Autodesk Inventor part; units mm, degrees
(part 2 of 2)
sketch "Sketch2" plane through (0, 0, 0.5) normal (0, 0, 1) x (1, 0, 0)
  line L0 (260.2818, -61.0161) -> (260.2818, -88.6954) projected
  line L1 (260.2818, -88.6954) -> (269.6798, -88.6954) projected
  line L2 (269.6798, -88.6954) -> (269.6798, -107.7454) projected
  line L3 (269.6798, -107.7454) -> (274.7598, -107.7454) projected
  line L4 (274.7598, -107.7454) -> (274.7598, -126.7954) projected
  line L5 (274.7598, -126.7954) -> (265.1048, -126.7954) projected
  line L6 (265.1048, -126.7954) -> (265.1048, -148.1602) projected
  line L7 (265.1048, -148.1602) -> (272.1064, -148.1602) projected
  line L8 (272.1064, -148.1602) -> (272.1064, -165) projected
  line L9 (272.1064, -165) -> (327.9413, -165) projected
  line L10 (327.9413, -165) -> (327.9413, -146) construction
  line L11 (327.9413, -146) -> (405.2108, -146) projected
  line L12 (405.2108, -146) -> (405.2108, -165) projected
  line L13 (405.2108, -165) -> (490, -165) projected
  line L14 (490, -165) -> (490, -69.6056) projected
  line L15 (490, -69.6056) -> (316.8693, -69.6056) projected
  line L16 (316.8693, -69.6056) -> (316.8693, -40) construction
  line L17 (316.8693, -40) -> (269.5528, -40) construction
  line L18 (269.5528, -40) -> (269.5528, -61.0161) construction
  line L19 (269.5528, -61.0161) -> (260.2818, -61.0161) projected
  line L20 (318.1433, -116.8724) -> (330.6708, -116.8724) projected
  line L21 (330.6708, -116.8724) -> (330.6708, -122.8724) projected
  line L22 (330.6708, -122.8724) -> (318.1433, -122.8724) projected
  line L23 (318.1433, -122.8724) -> (318.1433, -120.8724) projected
  line L24 (318.1433, -120.8724) -> (316.6433, -120.8724) projected
  line L25 (316.6433, -120.8724) -> (316.6433, -118.8724) projected
  line L26 (316.6433, -118.8724) -> (318.1433, -118.8724) projected
  line L27 (318.1433, -118.8724) -> (318.1433, -116.8724) projected
  line L28 (471.9563, -154.774) -> (484.4563, -154.774) projected
  line L29 (484.4563, -154.774) -> (484.4563, -160.774) projected
  line L30 (484.4563, -160.774) -> (471.9563, -160.774) projected
  line L31 (471.9563, -160.774) -> (471.9563, -158.774) projected
  line L32 (471.9563, -158.774) -> (470.4563, -158.774) projected
  line L33 (470.4563, -158.774) -> (470.4563, -156.774) projected
  line L34 (470.4563, -156.774) -> (471.9563, -156.774) projected
  line L35 (471.9563, -156.774) -> (471.9563, -154.774) projected
  line L36 (318.1433, -92.8724) -> (330.6708, -92.8724) projected
  line L37 (330.6708, -92.8724) -> (330.6708, -98.8724) projected
  line L38 (330.6708, -98.8724) -> (318.1433, -98.8724) projected
  line L39 (318.1433, -98.8724) -> (318.1433, -96.8724) projected
  line L40 (318.1433, -96.8724) -> (316.6433, -96.8724) projected
  line L41 (316.6433, -96.8724) -> (316.6433, -94.8724) projected
  line L42 (316.6433, -94.8724) -> (318.1433, -94.8724) projected
  line L43 (318.1433, -94.8724) -> (318.1433, -92.8724) projected
  circle A0 centre (265, -64.8616) radius 3.25 projected
  line L44 (471.7063, -138.7715) -> (485.7113, -138.7715) projected
  line L45 (485.7113, -138.7715) -> (485.7113, -152.7765) projected
  line L46 (485.7113, -152.7765) -> (471.7063, -152.7765) projected
  line L47 (471.7063, -152.7765) -> (471.7063, -138.7715) projected
  line L48 (452.6563, -148.3679) -> (466.6613, -148.3679) projected
  line L49 (466.6613, -148.3679) -> (466.6613, -162.3729) projected
  line L50 (466.6613, -162.3729) -> (452.6563, -162.3729) projected
  line L51 (452.6563, -162.3729) -> (452.6563, -148.3679) projected
  line L52 (424.2083, -148.3679) -> (438.2133, -148.3679) projected
  line L53 (438.2133, -148.3679) -> (438.2133, -162.3729) projected
  line L54 (438.2133, -162.3729) -> (424.2083, -162.3729) projected
  line L55 (424.2083, -162.3729) -> (424.2083, -148.3679) projected
  line L56 (452.6563, -129.2195) -> (466.6613, -129.2195) projected
  line L57 (466.6613, -129.2195) -> (466.6613, -143.2245) projected
  line L58 (466.6613, -143.2245) -> (452.6563, -143.2245) projected
  line L59 (452.6563, -143.2245) -> (452.6563, -129.2195) projected
  line L60 (433.6063, -129.2195) -> (447.6113, -129.2195) projected
  line L61 (447.6113, -129.2195) -> (447.6113, -143.2245) projected
  line L62 (447.6113, -143.2245) -> (433.6063, -143.2245) projected
  line L63 (433.6063, -143.2245) -> (433.6063, -129.2195) projected
  line L64 (414.5563, -129.2195) -> (428.5613, -129.2195) projected
  line L65 (428.5613, -129.2195) -> (428.5613, -143.2245) projected
  line L66 (428.5613, -143.2245) -> (414.5563, -143.2245) projected
  line L67 (414.5563, -143.2245) -> (414.5563, -129.2195) projected
  line L68 (452.6563, -110.1695) -> (466.6613, -110.1695) projected
  line L69 (466.6613, -110.1695) -> (466.6613, -124.1745) projected
  line L70 (466.6613, -124.1745) -> (452.6563, -124.1745) projected
  line L71 (452.6563, -124.1745) -> (452.6563, -110.1695) projected
  line L72 (433.6063, -110.1695) -> (447.6113, -110.1695) projected
  line L73 (447.6113, -110.1695) -> (447.6113, -124.1745) projected
  line L74 (447.6113, -124.1745) -> (433.6063, -124.1745) projected
  line L75 (433.6063, -124.1745) -> (433.6063, -110.1695) projected
  line L76 (414.5563, -110.1695) -> (428.5613, -110.1695) projected
  line L77 (428.5613, -110.1695) -> (428.5613, -124.1745) projected
  line L78 (428.5613, -124.1745) -> (414.5563, -124.1745) projected
  line L79 (414.5563, -124.1745) -> (414.5563, -110.1695) projected
  line L80 (414.5563, -91.1195) -> (428.5613, -91.1195) projected
  line L81 (428.5613, -91.1195) -> (428.5613, -105.1245) projected
  line L82 (428.5613, -105.1245) -> (414.5563, -105.1245) projected
  line L83 (414.5563, -105.1245) -> (414.5563, -91.1195) projected
  line L84 (433.6063, -91.1195) -> (447.6113, -91.1195) projected
  line L85 (447.6113, -91.1195) -> (447.6113, -105.1245) projected
  line L86 (447.6113, -105.1245) -> (433.6063, -105.1245) projected
  line L87 (433.6063, -105.1245) -> (433.6063, -91.1195) projected
  line L88 (452.6563, -91.1195) -> (466.6613, -91.1195) projected
  line L89 (466.6613, -91.1195) -> (466.6613, -105.1245) projected
  line L90 (466.6613, -105.1245) -> (452.6563, -105.1245) projected
  line L91 (452.6563, -105.1245) -> (452.6563, -91.1195) projected
  line L92 (471.7063, -91.1195) -> (485.7113, -91.1195) projected
  line L93 (485.7113, -91.1195) -> (485.7113, -105.1245) projected
  line L94 (485.7113, -105.1245) -> (471.7063, -105.1245) projected
  line L95 (471.7063, -105.1245) -> (471.7063, -91.1195) projected
  line L96 (471.7063, -72.0695) -> (485.7113, -72.0695) projected
  line L97 (485.7113, -72.0695) -> (485.7113, -86.0745) projected
  line L98 (485.7113, -86.0745) -> (471.7063, -86.0745) projected
  line L99 (471.7063, -86.0745) -> (471.7063, -72.0695) projected
  line L100 (452.6563, -72.0695) -> (466.6613, -72.0695) projected
  line L101 (466.6613, -72.0695) -> (466.6613, -86.0745) projected
  line L102 (466.6613, -86.0745) -> (452.6563, -86.0745) projected
  line L103 (452.6563, -86.0745) -> (452.6563, -72.0695) projected
  line L104 (433.6063, -72.0695) -> (447.6113, -72.0695) projected
  line L105 (447.6113, -72.0695) -> (447.6113, -86.0745) projected
  line L106 (447.6113, -86.0745) -> (433.6063, -86.0745) projected
  line L107 (433.6063, -86.0745) -> (433.6063, -72.0695) projected
  line L108 (414.5563, -72.0695) -> (428.5613, -72.0695) projected
  line L109 (428.5613, -72.0695) -> (428.5613, -86.0745) projected
  line L110 (428.5613, -86.0745) -> (414.5563, -86.0745) projected
  line L111 (414.5563, -86.0745) -> (414.5563, -72.0695) projected
  line L112 (381.1515, -72.1031) -> (395.1565, -72.1031) projected
  line L113 (395.1565, -72.1031) -> (395.1565, -86.1081) projected
  line L114 (395.1565, -86.1081) -> (381.1515, -86.1081) projected
  line L115 (381.1515, -86.1081) -> (381.1515, -72.1031) projected
  line L116 (352.5555, -72.1031) -> (366.5605, -72.1031) projected
  line L117 (366.5605, -72.1031) -> (366.5605, -86.1081) projected
  line L118 (366.5605, -86.1081) -> (352.5555, -86.1081) projected
  line L119 (352.5555, -86.1081) -> (352.5555, -72.1031) projected
  line L120 (366.8775, -110.2171) -> (380.8825, -110.2171) projected
  line L121 (380.8825, -110.2171) -> (380.8825, -124.2221) projected
  line L122 (380.8825, -124.2221) -> (366.8775, -124.2221) projected
  line L123 (366.8775, -124.2221) -> (366.8775, -110.2171) projected
  line L124 (385.9275, -129.2671) -> (399.9325, -129.2671) projected
  line L125 (399.9325, -129.2671) -> (399.9325, -143.2721) projected
  line L126 (399.9325, -143.2721) -> (385.9275, -143.2721) projected
  line L127 (385.9275, -143.2721) -> (385.9275, -129.2671) projected
  line L128 (366.8775, -129.2671) -> (380.8825, -129.2671) projected
  line L129 (380.8825, -129.2671) -> (380.8825, -143.2721) projected
  line L130 (380.8825, -143.2721) -> (366.8775, -143.2721) projected
  line L131 (366.8775, -143.2721) -> (366.8775, -129.2671) projected
  line L132 (347.8275, -129.2671) -> (361.8325, -129.2671) projected
  line L133 (361.8325, -129.2671) -> (361.8325, -143.2721) projected
  line L134 (361.8325, -143.2721) -> (347.8275, -143.2721) projected
  line L135 (347.8275, -143.2721) -> (347.8275, -129.2671) projected
  line L136 (302.9363, -148.3679) -> (316.9413, -148.3679) projected
  line L137 (316.9413, -148.3679) -> (316.9413, -162.3729) projected
  line L138 (316.9413, -162.3729) -> (302.9363, -162.3729) projected
  line L139 (302.9363, -162.3729) -> (302.9363, -148.3679) projected
  line L140 (279.0603, -148.3679) -> (293.0653, -148.3679) projected
  line L141 (293.0653, -148.3679) -> (293.0653, -162.3729) projected
  line L142 (293.0653, -162.3729) -> (279.0603, -162.3729) projected
  line L143 (279.0603, -162.3729) -> (279.0603, -148.3679) projected
  line L144 (303.4443, -129.3179) -> (317.4493, -129.3179) projected
  line L145 (317.4493, -129.3179) -> (317.4493, -143.3229) projected
  line L146 (317.4493, -143.3229) -> (303.4443, -143.3229) projected
  line L147 (303.4443, -143.3229) -> (303.4443, -129.3179) projected
  line L148 (267.6303, -129.3179) -> (281.6353, -129.3179) projected
  line L149 (281.6353, -129.3179) -> (281.6353, -143.3229) projected
  line L150 (281.6353, -143.3229) -> (267.6303, -143.3229) projected
  line L151 (267.6303, -143.3229) -> (267.6303, -129.3179) projected
  line L152 (296.3323, -110.2679) -> (310.3373, -110.2679) projected
  line L153 (310.3373, -110.2679) -> (310.3373, -124.2729) projected
  line L154 (310.3373, -124.2729) -> (296.3323, -124.2729) projected
  line L155 (296.3323, -124.2729) -> (296.3323, -110.2679) projected
  line L156 (277.2823, -110.2679) -> (291.2873, -110.2679) projected
  line L157 (291.2873, -110.2679) -> (291.2873, -124.2729) projected
  line L158 (291.2873, -124.2729) -> (277.2823, -124.2729) projected
  line L159 (277.2823, -124.2729) -> (277.2823, -110.2679) projected
  line L160 (317.6433, -100.8949) -> (331.6483, -100.8949) projected
  line L161 (331.6483, -100.8949) -> (331.6483, -114.8999) projected
  line L162 (331.6483, -114.8999) -> (317.6433, -114.8999) projected
  line L163 (317.6433, -114.8999) -> (317.6433, -100.8949) projected
  line L164 (291.2523, -91.2179) -> (305.2573, -91.2179) projected
  line L165 (305.2573, -91.2179) -> (305.2573, -105.2229) projected
  line L166 (305.2573, -105.2229) -> (291.2523, -105.2229) projected
  line L167 (291.2523, -105.2229) -> (291.2523, -91.2179) projected
  line L168 (272.2023, -91.2179) -> (286.2073, -91.2179) projected
  line L169 (286.2073, -91.2179) -> (286.2073, -105.2229) projected
  line L170 (286.2073, -105.2229) -> (272.2023, -105.2229) projected
  line L171 (272.2023, -105.2229) -> (272.2023, -91.2179) projected
  line L172 (319.9543, -72.1679) -> (333.9593, -72.1679) projected
  line L173 (333.9593, -72.1679) -> (333.9593, -86.1729) projected
  line L174 (333.9593, -86.1729) -> (319.9543, -86.1729) projected
  line L175 (319.9543, -86.1729) -> (319.9543, -72.1679) projected
  line L176 (300.9043, -72.1679) -> (314.9093, -72.1679) projected
  line L177 (314.9093, -72.1679) -> (314.9093, -86.1729) projected
  line L178 (314.9093, -86.1729) -> (300.9043, -86.1729) projected
  line L179 (300.9043, -86.1729) -> (300.9043, -72.1679) projected
  line L180 (281.8543, -72.1679) -> (295.8593, -72.1679) projected
  line L181 (295.8593, -72.1679) -> (295.8593, -86.1729) projected
  line L182 (295.8593, -86.1729) -> (281.8543, -86.1729) projected
  line L183 (281.8543, -86.1729) -> (281.8543, -72.1679) projected
  line L184 (262.8043, -72.1679) -> (276.8093, -72.1679) projected
  line L185 (276.8093, -72.1679) -> (276.8093, -86.1729) projected
  line L186 (276.8093, -86.1729) -> (262.8043, -86.1729) projected
  line L187 (262.8043, -86.1729) -> (262.8043, -72.1679) projected
  line L188 (298.3643, -43.5111) -> (312.3693, -43.5111) projected
  line L189 (312.3693, -43.5111) -> (312.3693, -57.5161) projected
  line L190 (312.3693, -57.5161) -> (298.3643, -57.5161) projected
  line L191 (298.3643, -57.5161) -> (298.3643, -43.5111) projected
  line L192 (274.4883, -43.5111) -> (288.4933, -43.5111) projected
  line L193 (288.4933, -43.5111) -> (288.4933, -57.5161) projected
  line L194 (288.4933, -57.5161) -> (274.4883, -57.5161) projected
  line L195 (274.4883, -57.5161) -> (274.4883, -43.5111) projected
  line L196 (471.9563, -130.774) -> (484.4563, -130.774) projected
  line L197 (484.4563, -130.774) -> (484.4563, -136.774) projected
  line L198 (484.4563, -136.774) -> (471.9563, -136.774) projected
  line L199 (471.9563, -136.774) -> (471.9563, -134.774) projected
  line L200 (471.9563, -134.774) -> (470.4563, -134.774) projected
  line L201 (470.4563, -134.774) -> (470.4563, -132.774) projected
  line L202 (470.4563, -132.774) -> (471.9563, -132.774) projected
  line L203 (471.9563, -132.774) -> (471.9563, -130.774) projected
  line L204 (446.2108, -148.6179) -> (446.2108, -161.1179) projected
  line L205 (446.2108, -161.1179) -> (440.2108, -161.1179) projected
  line L206 (440.2108, -161.1179) -> (440.2108, -148.6179) projected
  line L207 (440.2108, -148.6179) -> (442.2108, -148.6179) projected
  line L208 (442.2108, -148.6179) -> (442.2108, -147.1179) projected
  line L209 (442.2108, -147.1179) -> (444.2108, -147.1179) projected
  line L210 (444.2108, -147.1179) -> (444.2108, -148.6179) projected
  line L211 (444.2108, -148.6179) -> (446.2108, -148.6179) projected
  line L212 (422.2108, -148.6179) -> (422.2108, -161.1179) projected
  line L213 (422.2108, -161.1179) -> (416.2108, -161.1179) projected
  line L214 (416.2108, -161.1179) -> (416.2108, -148.6179) projected
  line L215 (416.2108, -148.6179) -> (418.2108, -148.6179) projected
  line L216 (418.2108, -148.6179) -> (418.2108, -147.1179) projected
  line L217 (418.2108, -147.1179) -> (420.2108, -147.1179) projected
  line L218 (420.2108, -147.1179) -> (420.2108, -148.6179) projected
  line L219 (420.2108, -148.6179) -> (422.2108, -148.6179) projected
  line L220 (325.4468, -129.8179) -> (325.4468, -142.3179) projected
  line L221 (325.4468, -142.3179) -> (319.4468, -142.3179) projected
  line L222 (319.4468, -142.3179) -> (319.4468, -129.8179) projected
  line L223 (319.4468, -129.8179) -> (321.4468, -129.8179) projected
  line L224 (321.4468, -129.8179) -> (321.4468, -128.3179) projected
  line L225 (321.4468, -128.3179) -> (323.4468, -128.3179) projected
  line L226 (323.4468, -128.3179) -> (323.4468, -129.8179) projected
  line L227 (323.4468, -129.8179) -> (325.4468, -129.8179) projected
  line L228 (301.4468, -129.8179) -> (301.4468, -142.3179) projected
  line L229 (301.4468, -142.3179) -> (295.4468, -142.3179) projected
  line L230 (295.4468, -142.3179) -> (295.4468, -129.8179) projected
  line L231 (295.4468, -129.8179) -> (297.4468, -129.8179) projected
  line L232 (297.4468, -129.8179) -> (297.4468, -128.3179) projected
  line L233 (297.4468, -128.3179) -> (299.4468, -128.3179) projected
  line L234 (299.4468, -128.3179) -> (299.4468, -129.8179) projected
  line L235 (299.4468, -129.8179) -> (301.4468, -129.8179) projected
  line L236 (471.7063, -110.1695) -> (485.7113, -110.1695) projected
  line L237 (485.7113, -110.1695) -> (485.7113, -123.8288) projected
  arc A1 (483.3941, -124.1745) -> (485.7113, -123.8288) centre (485, -127) ccw projected
  line L238 (483.3941, -124.1745) -> (471.7063, -124.1745) projected
  line L239 (471.7063, -124.1745) -> (471.7063, -110.1695) projected
  line L240 (412.0563, -69.6056) -> (412.0563, -165)
  line L241 (327.9413, -146) -> (405.2108, -146) projected
  line L242 (345.33, -146) -> (345.33, -126.7696)
  line L243 (345.33, -126.7696) -> (364.38, -126.7696)
  line L244 (364.38, -126.7696) -> (364.38, -107.7196)
  line L245 (364.38, -107.7196) -> (383.38, -107.7196)
  line L246 (383.38, -107.7196) -> (383.38, -126.7696)
  line L247 (383.38, -126.7696) -> (402.43, -126.7696)
  line L248 (402.43, -126.7696) -> (402.43, -146)
  line L249 (345.5555, -69.6056) -> (345.5555, -88.6056)
  line L250 (345.5555, -88.6056) -> (402.1565, -88.6056)
  line L251 (402.1565, -88.6056) -> (402.1565, -69.6056)
  line L252 (490, -69.6056) -> (316.8693, -69.6056) projected
  line L253 (336.4593, -146) -> (336.4593, -69.6056)
  line L254 (316.8693, -69.6056) -> (260.2818, -69.6056)
  circle A2 centre (281.4908, -50.5136) radius 2.55 construction
  line L255 (269.5528, -60.0136) -> (316.8693, -60.0136)
  line L256 (269.5528, -41.0136) -> (316.8693, -41.0136)
  line L257 (269.5528, -40) -> (269.5528, -61.0161) projected
  line L258 (269.5528, -41.0136) -> (269.5528, -61.0161)
  line L259 (316.8693, -69.6056) -> (316.8693, -40) projected
  line L260 (316.8693, -41.0136) -> (316.8693, -69.6056)
  line L261 (322.4388, -165) -> (322.4388, -146)
  line L262 (322.4388, -146) -> (327.9413, -146)
  circle A3 centre (309.9388, -155.3704) radius 2.55 construction
  line L263 (490, -69.6056) -> (316.8693, -69.6056) projected
  line L264 (488.7088, -69.6056) -> (488.7088, -165)
  circle A4 centre (478.7088, -79.072) radius 2.55 projected
  circle A5 centre (359.558, -79.1056) radius 2.55 projected
  circle A6 centre (373.88, -117.2196) radius 2.55 projected
  circle A7 centre (354.83, -136.2696) radius 2.55 projected
  circle A8 centre (392.93, -136.2696) radius 2.55 projected
  point P0 (0, 0)
  point P1 (316.8693, -61.0161)
  point P2 (402.1565, -69.6056)
  point P3 (336.4593, -69.6056)
  dimension "d103" = 7
  dimension "d104" = 7
  dimension "d106" = 2.5
  dimension "d113" = 2.5
  dimension "d118" = 9.5
  dimension "d133" = 9.5
  dimension "d134" = 12.5
  dimension "d135" = 10
  dimension "d136" = 9.5
  dimension "d137" = 9.5
  dimension "d138" = 9.5
  dimension "d139" = 9.5
  dimension "d140" = 9.5
  dimension "d141" = 9.5
  dimension "d142" = 9.5
  constraints: 40 end point, 19 point on line, 17 perpendicular, 1 collinear, 1 vertical
  measures "d103" distance between parallel lines of L119 L249
  measures "d104" distance between parallel lines of L251 L113
  measures "d106" distance between parallel lines of L253 L173
  measures "d113" distance between parallel lines of L111 L240
  measures "d118" distance from line of L255 A2.centre
  measures "d133" distance from line of L256 A2.centre
  measures "d134" distance from line of L261 A3.centre
  measures "d135" distance from line of L264 A4.centre
  measures "d136" distance from line of L250 A5.centre
  measures "d137" distance from line of L242 A7.centre
  measures "d138" distance from line of L243 A7.centre
  measures "d139" distance from line of L248 A8.centre
  measures "d140" distance from line of L244 A6.centre
  measures "d141" distance from line of L245 A6.centre
  measures "d142" distance from line of L246 A6.centre
extrude "Extrusion4" add sketch "Sketch2" along normal blind 2.5 contours L254 L15 L253 L11 L262 L261 L9 L8 L7 L6 L5 L4 L3 L2 L1 L0 | L257 L256 L259 L255 | L15 L251 L250 L249 | L242 L243 L244 L245 L246 L247 L248 L11 | L15 L264 L13 L240
sketch "Sketch3" plane through (0, 0, 0) normal (0, 0, -1) x (-1, 0, 0)
  line L0 (-485.7063, -130.774) -> (-468.7063, -130.774)
  line L1 (-471.9563, -130.774) -> (-484.4563, -130.774) projected
  line L2 (-468.7063, -130.774) -> (-468.7063, -160.774)
  line L3 (-468.7063, -160.774) -> (-485.7063, -160.774)
  line L4 (-485.7063, -160.774) -> (-485.7063, -154.774)
  line L5 (-485.7063, -154.774) -> (-475.2063, -154.774)
  line L6 (-471.9563, -154.774) -> (-484.4563, -154.774) projected
  line L7 (-475.2063, -154.774) -> (-475.2063, -136.774)
  line L8 (-484.4563, -136.774) -> (-471.9563, -136.774) projected
  line L9 (-475.2063, -136.774) -> (-485.7063, -136.774)
  line L10 (-485.7063, -136.774) -> (-485.7063, -130.774)
  line L11 (-471.7063, -152.7765) -> (-471.7063, -138.7715) projected
  line L12 (-484.4563, -160.774) -> (-471.9563, -160.774) projected
  line L13 (-446.2108, -162.3679) -> (-446.2108, -145.3679)
  line L14 (-446.2108, -145.3679) -> (-416.2108, -145.3679)
  line L15 (-416.2108, -148.6179) -> (-418.2108, -148.6179) projected
  line L16 (-416.2108, -145.3679) -> (-416.2108, -162.3679)
  line L17 (-416.2108, -162.3679) -> (-422.2108, -162.3679)
  line L18 (-422.2108, -162.3679) -> (-422.2108, -151.8679)
  line L19 (-422.2108, -148.6179) -> (-422.2108, -161.1179) projected
  line L20 (-440.2108, -161.1179) -> (-440.2108, -148.6179) projected
  line L21 (-440.2108, -151.8679) -> (-422.2108, -151.8679)
  line L22 (-440.2108, -151.8679) -> (-440.2108, -162.3679)
  line L23 (-440.2108, -162.3679) -> (-446.2108, -162.3679)
  line L24 (-424.2083, -148.3679) -> (-438.2133, -148.3679) projected
  line L25 (-446.2108, -148.6179) -> (-446.2108, -161.1179) projected
  line L26 (-416.2108, -161.1179) -> (-416.2108, -148.6179) projected
  line L27 (-422.2108, -148.6179) -> (-422.2108, -161.1179) projected
  line L28 (-331.6433, -92.8724) -> (-314.6433, -92.8724)
  line L29 (-318.1433, -92.8724) -> (-330.6708, -92.8724) projected
  line L30 (-314.6433, -92.8724) -> (-314.6433, -122.8724)
  line L31 (-314.6433, -122.8724) -> (-331.6433, -122.8724)
  line L32 (-331.6433, -122.8724) -> (-331.6433, -116.8724)
  line L33 (-331.6433, -116.8724) -> (-321.1433, -116.8724)
  line L34 (-318.1433, -116.8724) -> (-330.6708, -116.8724) projected
  line L35 (-321.1433, -116.8724) -> (-321.1433, -98.8724)
  line L36 (-321.1433, -98.8724) -> (-331.6433, -98.8724)
  line L37 (-331.6433, -98.8724) -> (-331.6433, -92.8724)
  line L38 (-317.6433, -114.8999) -> (-317.6433, -100.8949) projected
  line L39 (-330.6708, -98.8724) -> (-318.1433, -98.8724) projected
  line L40 (-330.6708, -122.8724) -> (-318.1433, -122.8724) projected
  line L41 (-325.4468, -143.3179) -> (-325.4468, -126.3179)
  line L42 (-325.4468, -126.3179) -> (-295.4468, -126.3179)
  line L43 (-295.4468, -126.3179) -> (-295.4468, -143.3179)
  line L44 (-295.4468, -142.3179) -> (-295.4468, -129.8179) projected
  line L45 (-295.4468, -143.3179) -> (-301.4468, -143.3179)
  line L46 (-301.4468, -143.3179) -> (-301.4468, -132.8179)
  line L47 (-301.4468, -129.8179) -> (-301.4468, -142.3179) projected
  line L48 (-319.4468, -142.3179) -> (-319.4468, -129.8179) projected
  line L49 (-319.4468, -132.8179) -> (-301.4468, -132.8179)
  line L50 (-319.4468, -132.8179) -> (-319.4468, -143.3179)
  line L51 (-319.4468, -143.3179) -> (-325.4468, -143.3179)
  line L52 (-303.4443, -129.3179) -> (-317.4493, -129.3179) projected
  line L53 (-325.4468, -129.8179) -> (-325.4468, -142.3179) projected
  point P0 (0, 0)
  dimension "d119" = 17
  dimension "d120" = 3
  dimension "d121" = 3.5
  dimension "d122" = 3.5
  dimension "d123" = 3
  dimension "d124" = 17
  dimension "d125" = 3
  dimension "d126" = 3.5
  dimension "d127" = 17
  dimension "d128" = 3
  dimension "d129" = 3.5
  dimension "d130" = 17
  constraints: 64 end point, 20 perpendicular, 16 collinear, 11 point on line, 3 vertical, 1 parallel
  measures "d119" distance between parallel lines of L2 L10
  measures "d120" distance between parallel lines of L2 L11
  measures "d121" distance between parallel lines of L11 L7
  measures "d122" distance between parallel lines of L21 L24
  measures "d123" distance between parallel lines of L14 L24
  measures "d124" distance of L13.start L13.end
  measures "d125" distance between parallel lines of L30 L38
  measures "d126" distance between parallel lines of L38 L35
  measures "d127" distance between parallel lines of L30 L37
  measures "d128" distance between parallel lines of L42 L52
  measures "d129" distance between parallel lines of L49 L52
  measures "d130" distance between parallel lines of L51 L42
extrude "Extrusion5" cut sketch "Sketch3" against normal blind 2
sketch "Sketch4" plane through (269.5528, -61.0161, 0) normal (-1, 0, 0) x (0, 0, 1)
  line L0 (0, 21.0161) -> (0, 0) projected
  line L1 (0.5, 1.0025) -> (3, 1.0025) projected
  line L2 (0, 20.0025) -> (1.4, 20.0025)
  line L3 (1.4, 20.0025) -> (1.4, 1.0025)
  line L4 (1.4, 1.0025) -> (0, 1.0025)
  line L5 (0, 1.0025) -> (0, 20.0025)
  line L6 (0.5, 20.0025) -> (3, 20.0025) projected
  point P0 (0, 61.0161)
  dimension "d147" = 1.4
  constraints: 8 end point, 2 parallel, 2 point on line, 1 collinear, 1 horizontal, 1 perpendicular
  measures "d147" distance of L3.end L4.end
extrude "underlap 1" add sketch "Sketch4" along normal blind 2
sketch "Sketch5" plane through (269.6798, -107.7454, 0) normal (-1, 0, 0) x (0, 0, 1)
  line L0 (0, 19.05) -> (0, 0) projected
  line L1 (0, 0) -> (3, 0) projected
  line L2 (0, 19.05) -> (1.4, 19.05)
  line L3 (1.4, 19.05) -> (1.4, 0)
  line L4 (1.4, 0) -> (0, 0)
  line L5 (0, 0) -> (0, 19.05)
  point P0 (0, 107.7454)
  dimension "d150" = 1.4
  constraints: 8 end point, 2 parallel, 1 horizontal, 1 perpendicular, 1 point on line
  measures "d150" distance of L3.end L4.end
extrude "underlap 3" add sketch "Sketch5" along normal blind 2
sketch "Sketch6" plane through (265.1048, -148.1602, 0) normal (-1, 0, 0) x (0, 0, 1)
  line L0 (0, 0) -> (3, 0) projected
  line L1 (0, 21.3648) -> (1.4, 21.3648)
  line L2 (1.4, 21.3648) -> (1.4, 0)
  line L3 (1.4, 0) -> (0, 0)
  line L4 (0, 0) -> (0, 21.3648)
  point P0 (0, 148.1602)
  dimension "d153" = 1.4
  constraints: 8 end point, 2 parallel, 1 horizontal, 1 perpendicular, 1 point on line
  measures "d153" distance of L2.end L3.end
extrude "underlap 5" add sketch "Sketch6" along normal blind 2
sketch "Sketch7" plane through (272.1064, -165, 0) normal (-1, 0, 0) x (0, 0, 1)
  line L0 (0, 16.8398) -> (3, 16.8398) projected
  line L1 (0, 0) -> (3, 0) projected
  line L2 (3, 16.8398) -> (1.5, 16.8398)
  line L3 (1.5, 16.8398) -> (1.5, 0)
  line L4 (1.5, 0) -> (3, 0)
  line L5 (3, 0) -> (3, 16.8398)
  point P0 (0, 165)
  point P1 (1.5, 16.8398)
  constraints: 8 end point, 2 parallel, 1 horizontal, 1 midpoint, 1 perpendicular
extrude "overlap 6" add sketch "Sketch7" along normal blind 2
sketch "Sketch8" plane through (274.7598, -126.7954, 0) normal (-1, 0, 0) x (0, 0, 1)
  line L0 (3, 19.05) -> (3, 0) projected
  line L1 (0, 0) -> (3, 0) projected
  line L2 (3, 19.05) -> (1.5, 19.05)
  line L3 (1.5, 19.05) -> (1.5, 0)
  line L4 (1.5, 0) -> (3, 0)
  line L5 (3, 0) -> (3, 19.05)
  point P0 (0, 126.7954)
  constraints: 8 end point, 2 parallel, 1 horizontal, 1 midpoint, 1 perpendicular
extrude "overlap 4" add sketch "Sketch8" along normal blind 2
sketch "Sketch9" plane through (260.2818, -88.6954, 0) normal (-1, 0, 0) x (0, 0, 1)
  line L0 (3, 19.0898) -> (3, 0) projected
  line L1 (0.5, 19.0898) -> (3, 19.0898) projected
  line L2 (3, 0) -> (1.5, 0)
  line L3 (1.5, 0) -> (1.5, 19.0898)
  line L4 (1.5, 19.0898) -> (3, 19.0898)
  line L5 (3, 19.0898) -> (3, 0)
  point P0 (0, 88.6954)
  dimension "d160" = 1.5
  constraints: 8 end point, 2 parallel, 1 horizontal, 1 perpendicular, 1 point on line
  measures "d160" distance of L3.end L4.end
extrude "overlap 2" add sketch "Sketch9" along normal blind 2
sketch "Sketch10" plane through (0, 0, 3) normal (0, 0, 1) x (1, 0, 0)
  line L0 (350.1187, -113.568) -> (357.0109, -113.568) construction
  line L1 (357.0109, -113.568) -> (357.0109, -116.6585) construction
  line L2 (357.0109, -116.6585) -> (350.1187, -116.6585) construction
  line L3 (350.1187, -116.6585) -> (350.1187, -113.568) construction
  line L4 (353.3332, -113.568) -> (351.9208, -116.6585)
  line L5 (351.9208, -116.6585) -> (351.5918, -116.6585)
  line L6 (351.5918, -116.6585) -> (350.1187, -113.568)
  line L7 (350.1187, -113.568) -> (350.9464, -113.568)
  line L8 (350.9464, -113.568) -> (351.7513, -115.3094)
  line L9 (351.7513, -115.3094) -> (352.5157, -113.568)
  line L10 (352.5157, -113.568) -> (353.3332, -113.568)
  point P0 (0, 0)
  constraints: 2 other
extrude "Extrusion12" add sketch "Sketch10" along normal blind 0.5
equation "\"d0\" = sw"
equation "\"d1\" = sw"
equation "\"d2\" = sw"
equation "\"d3\" = sw"
equation "\"d4\" = sw"
equation "\"d5\" = sw"
equation "\"d6\" = sw"
equation "\"d7\" = sw"
equation "\"d8\" = sw"
equation "\"d9\" = sw"
equation "\"d10\" = sw"
equation "\"d11\" = sw"
equation "\"d12\" = sw"
equation "\"d13\" = sw"
equation "\"d14\" = sw"
equation "\"d15\" = sw"
equation "\"d16\" = sw"
equation "\"d17\" = sw"
equation "\"d18\" = sw"
equation "\"d19\" = sw"
equation "\"d20\" = sw"
equation "\"d21\" = sw"
equation "\"d22\" = sw"
equation "\"d23\" = sw"
equation "\"d24\" = sw"
equation "\"d25\" = sw"
equation "\"d26\" = sw"
equation "\"d27\" = sw"
equation "\"d28\" = sw"
equation "\"d29\" = sw"
equation "\"d30\" = sw"
equation "\"d31\" = sw"
equation "\"d32\" = sw"
equation "\"d33\" = sw"
equation "\"d34\" = sw"
equation "\"d35\" = sw"
equation "\"d36\" = sw"
equation "\"d37\" = sw"
equation "\"d38\" = sw"
equation "\"d39\" = sw"
equation "\"d40\" = sw"
equation "\"d41\" = sw"
equation "\"d42\" = sw"
equation "\"d43\" = sw"
equation "\"d44\" = sw"
equation "\"d45\" = sw"
equation "\"d46\" = sw"
equation "\"d47\" = sw"
equation "\"d48\" = sw"
equation "\"d49\" = sw"
equation "\"d50\" = sw"
equation "\"d51\" = sw"
equation "\"d52\" = sw"
equation "\"d53\" = sw"
equation "\"d54\" = sw"
equation "\"d55\" = sw"
equation "\"d56\" = sw"
equation "\"d57\" = sw"
equation "\"d58\" = sw"
equation "\"d59\" = sw"
equation "\"d60\" = sw"
equation "\"d61\" = sw"
equation "\"d62\" = sw"
equation "\"d63\" = sw"
equation "\"sw\" = 14.005"
body "Solid1"
